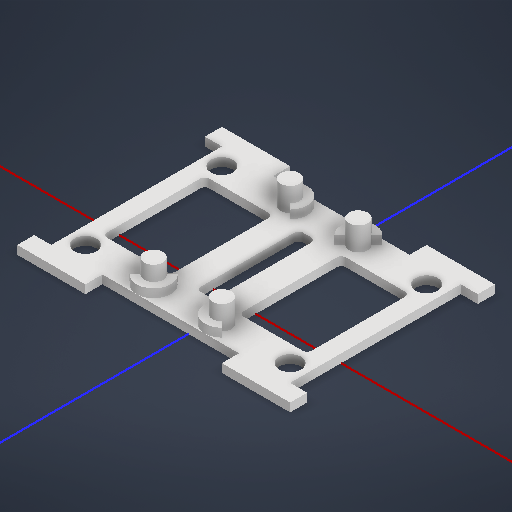
# Autodesk Inventor part: base
Saved by Autodesk Inventor 2025.4 (Build 294407000, 407)
## iProperties
Created: 2026-09-15
Part Number: base
Material: Generic
Document SubType Name: Sheet Metal
Designer: User
Density: 1 g/cm^3
Appearance: Default
Sheet Metal Rule: Default
Author: User
Autodesk Inventor part; units mm, degrees
ref_plane "YZ Plane" through (0, 0, 0) normal (1, 0, 0) x (0, 1, 0)
ref_plane "XZ Plane" through (0, 0, 0) normal (0, 1, 0) x (-1, 0, 0)
ref_plane "XY Plane" through (0, 0, 0) normal (0, 0, 1) x (1, 0, 0)
sketch "Sketch1" plane through (0, 0, 0) normal (0, 1, 0) x (-1, 0, 0)
  line L0 (-10, -14) -> (10, -14)
  line L1 (10, -14) -> (10, 14)
  line L2 (10, 14) -> (-10, 14)
  line L3 (-10, 14) -> (-10, -14)
  line L4 (-10, -14) -> (10, 14) construction
  line L5 (10, -14) -> (-10, 14) construction
  line L6 (-8, -4) -> (8, -4)
  line L7 (8, -4) -> (8, 4)
  line L8 (8, 4) -> (-8, 4)
  line L9 (-8, 4) -> (-8, -4)
  line L10 (-8, -4) -> (8, 4) construction
  line L11 (8, -4) -> (-8, 4) construction
  line L12 (-10, 8) -> (-12, 8)
  line L13 (-12, 8) -> (-12, 16)
  line L14 (-12, 16) -> (-10, 16)
  line L15 (-10, 16) -> (-10, 8)
  line L16 (10, 8) -> (12, 8)
  line L17 (12, 8) -> (12, 16)
  line L18 (12, 16) -> (10, 16)
  line L19 (10, 16) -> (10, 8)
  line L20 (10, -8) -> (12, -8)
  line L21 (12, -8) -> (12, -16)
  line L22 (12, -16) -> (10, -16)
  line L23 (10, -16) -> (10, -8)
  line L24 (-10, -8) -> (-12, -8)
  line L25 (-12, -8) -> (-12, -16)
  line L26 (-12, -16) -> (-10, -16)
  line L27 (-10, -16) -> (-10, -8)
  circle A0 centre (-8, 4) radius 2
  circle A1 centre (8, -4) radius 2
  circle A2 centre (-8, -4) radius 2
  circle A3 centre (8, 4) radius 2
  line L28 (5.5, -4) -> (-5.5, -4)
  line L29 (-6, -4.5) -> (-6, -11.5)
  line L30 (-5.5, -12) -> (5.5, -12)
  line L31 (6, -11.5) -> (6, -4.5)
  arc A4 (5.5, -12) -> (6, -11.5) centre (5.5, -11.5) ccw
  arc A5 (6, -4.5) -> (5.5, -4) centre (5.5, -4.5) ccw
  arc A6 (-6, -11.5) -> (-5.5, -12) centre (-5.5, -11.5) ccw
  arc A7 (-5.5, -4) -> (-6, -4.5) centre (-5.5, -4.5) ccw
  line L32 (5.5, 4) -> (-5.5, 4)
  line L33 (-6, 4.5) -> (-6, 11.5)
  line L34 (-5.5, 12) -> (5.5, 12)
  line L35 (6, 11.5) -> (6, 4.5)
  arc A8 (5.5, 4) -> (6, 4.5) centre (5.5, 4.5) ccw
  arc A9 (-6, 4.5) -> (-5.5, 4) centre (-5.5, 4.5) ccw
  arc A10 (6, 11.5) -> (5.5, 12) centre (5.5, 11.5) ccw
  arc A11 (-5.5, 12) -> (-6, 11.5) centre (-5.5, 11.5) ccw
  line L36 (5.5, 1) -> (-5.5, 1)
  line L37 (-6, 0.5) -> (-6, -0.5)
  line L38 (-5.5, -1) -> (5.5, -1)
  line L39 (6, -0.5) -> (6, 0.5)
  line L40 (6, 1) -> (-6, -1) construction
  line L41 (-6, 1) -> (6, -1) construction
  arc A12 (-5.5, 1) -> (-6, 0.5) centre (-5.5, 0.5) ccw
  arc A13 (-6, -0.5) -> (-5.5, -1) centre (-5.5, -0.5) ccw
  arc A14 (5.5, -1) -> (6, -0.5) centre (5.5, -0.5) ccw
  arc A15 (6, 0.5) -> (5.5, 1) centre (5.5, 0.5) ccw
  circle A16 centre (-8, 12) radius 1.3
  circle A17 centre (8, 12) radius 1.3
  circle A18 centre (-8, -12) radius 1.3
  circle A19 centre (8, -12) radius 1.3
  line L42 (-8.5858, -5.4142) -> (-4.5858, -5.4142) construction
  line L43 (11.4142, -2.5858) -> (15.4142, -2.5858) construction
  line L44 (11.4142, 2.5858) -> (15.4142, 2.5858) construction
  line L45 (-8.5858, 5.4142) -> (-4.5858, 5.4142) construction
  point P0 (0, 0)
  point P1 (-10, -14)
  point P2 (10, 4)
  point P3 (-10, 4)
  point P4 (-10, -4)
  point P5 (10, -4)
  point P6 (6, -4)
  point P7 (-6, -12)
  point P8 (-6, -4)
  point P9 (6, -12)
  point P10 (6, 4)
  point P11 (-6, 12)
  point P12 (-6, 4)
  point P13 (6, 12)
  point P14 (-5.5, 4)
  point P15 (-14.5, 16)
  point P16 (10.5, 16)
  point P17 (14.3, -16)
  point P18 (-12.7, -16)
  point P19 (12, -11)
  point P20 (12, 7)
  point P21 (-12, -6.8)
  point P22 (-12, 8.8)
  dimension "d45" = 4
  dimension "d47" = 4
  dimension "d0" = 20
  dimension "d1" = 28
  dimension "d2" = 16
  dimension "d3" = 8
  dimension "d33" = 8
  dimension "d34" = 2
  dimension "d37" = 2
  dimension "d38" = 2
  dimension "d40" = 2
  dimension "d43" = 2
  dimension "d44" = 4
  dimension "d46" = 4
  dimension "d54" = 12
  dimension "d55" = 8
  dimension "d56" = 0.5
  dimension "d57" = 12
  dimension "d58" = 8
  dimension "d59" = 0.5
  dimension "d60" = 0.5
  dimension "d61" = 12
  dimension "d62" = 2
  dimension "d63" = 0.5
  dimension "d93" = 2.6
  dimension "d94" = 2
  dimension "d96" = 2
  dimension "d97" = 2.6
  dimension "d98" = 2
  dimension "d99" = 2
  dimension "d100" = 2.6
  dimension "d101" = 2
  dimension "d102" = 2
  dimension "d103" = 2.6
  dimension "d104" = 2
  dimension "d105" = 2
  constraints: 92 end point, 38 point on line, 24 point on circle, 24 tangent, 18 centre point, 18 parallel, 13 horizontal, 9 perpendicular, 8 equal radius, 6 equal length, 6 midpoint, 4 coincident, 6 other
  measures "d0" distance of L2.end L1.end
  measures "d1" distance of L1.end L0.end
  measures "d2" distance of L8.end L7.end
  measures "d3" distance of L7.end L6.end
  measures "d33" distance of L12.end L13.end
  measures "d34" distance between parallel lines of L2 L14
  measures "d37" distance between parallel lines of L2 L18
  measures "d38" distance of L21.end L22.end
  measures "d40" distance between parallel lines of L0 L22
  measures "d43" distance between parallel lines of L0 L26
  measures "d44" diameter of A0
  measures "d46" diameter of A2
  measures "d54" distance of point (6, -12) point (-6, -12)
  measures "d55" distance of point (-6, -12) point (-6, -4)
  measures "d56" radius of A4
  measures "d57" distance of point (-6, 12) point (6, 12)
  measures "d58" distance of point (-6, 4) point (-6, 12)
  measures "d59" radius of A8
  measures "d60" radius of A10
  measures "d61" distance of L41.end L40.end
  measures "d62" distance of L40.end L41.start
  measures "d63" radius of A12
  measures "d93" diameter of A16
  measures "d94" distance from line of L2 A16.centre
  measures "d96" distance from line of L3 A16.centre
  measures "d97" diameter of A17
  measures "d98" distance from line of L2 A17.centre
  measures "d99" distance from line of L1 A17.centre
  measures "d100" diameter of A18
  measures "d101" distance from line of L3 A18.centre
  measures "d102" distance from line of L0 A18.centre
  measures "d103" diameter of A19
  measures "d104" distance from line of L1 A19.centre
  measures "d105" distance from line of L0 A19.centre
extrude "Extrusion1" add sketch "Sketch1" along normal blind 1 contours L3 A2 L6 A7 L29 A6 L30 A4 L31 A5 A1 L1 L0 | L27 L26 L25 L24 L3 | L1 L20 L21 L22 L23 | L3 A0 L9 A2 | A1 L7 A3 L1 | L3 L2 L1 A3 L8 A8 L35 A10 L34 A11 L33 A9 A0 | L9 A0 L8 A3 L7 A1 L6 A2 | L12 L13 L14 L15 L3 | L1 L19 L18 L17 L16
sketch "Sketch2" plane through (0, 0, 0) normal (0, -1, 0) x (1, 0, 0)
  line L0 (10, -14) -> (-10, -14) projected
  line L1 (10, -4) -> (10, -8) projected
  line L2 (-10, 14) -> (10, 14) projected
  line L3 (-12, -8) -> (-10, -8) projected
  line L4 (-12, -16) -> (-12, -8) projected
  line L5 (-10, -16) -> (-12, -16) projected
  line L6 (-10, 4) -> (-10, 8) projected
  line L7 (12, -16) -> (10, -16) projected
  line L8 (12, -8) -> (12, -16) projected
  line L9 (10, -8) -> (12, -8) projected
  line L10 (12, 8) -> (10, 8) projected
  line L11 (12, 16) -> (12, 8) projected
  line L12 (10, 16) -> (12, 16) projected
  line L13 (10, -16) -> (10, -14) projected
  line L14 (-10, 16) -> (-10, 14) projected
  line L15 (-12, 16) -> (-10, 16) projected
  line L16 (-12, 8) -> (-12, 16) projected
  line L17 (-10, 8) -> (-12, 8) projected
  circle A0 centre (-8, 4) radius 2 projected
  line L18 (-10, -4) -> (-10, 4) projected
  circle A1 centre (-8, -4) radius 2 projected
  line L19 (-10, -8) -> (-10, -4) projected
  circle A2 centre (8, -4) radius 2 projected
  line L20 (10, 4) -> (10, -4) projected
  circle A3 centre (8, 4) radius 2 projected
  line L21 (10, 8) -> (10, 4) projected
  line L22 (10, 14) -> (10, 16) projected
  line L23 (-10, -14) -> (-10, -16) projected
  point P0 (0, 0)
  constraints: 4 horizontal alignment
extrude "Extrusion2" add sketch "Sketch2" against normal blind 2 contours A2 | A3 | A0 | A1
sketch "Sketch3" plane through (8, 2, 4) normal (0, 1, 0) x (1, 0, 0)
  circle A0 centre (-16, 8) radius 2 projected
  circle A1 centre (0, 8) radius 2 projected
  circle A2 centre (0, 0) radius 2 projected
  circle A3 centre (-16, 0) radius 2 projected
  circle A4 centre (-16, 8) radius 1.1
  circle A5 centre (0, 8) radius 1.1
  circle A6 centre (0, 0) radius 1.1
  circle A7 centre (-16, 0) radius 1.1
  point P0 (-8, 4)
  dimension "d48" = 2.2
  dimension "d49" = 2.2
  dimension "d50" = 2.2
  dimension "d51" = 2.2
  constraints: 4 centre point, 4 coincident
  measures "d48" diameter of A4
  measures "d49" diameter of A5
  measures "d50" diameter of A6
  measures "d51" diameter of A7
extrude "Extrusion3" add sketch "Sketch3" along normal blind 1.75 contours A4 | A5 | A6 | A7
sketch "Sketch4" plane through (-8, 2, -4) normal (0, 1, 0) x (1, 0, 0)
  circle A0 centre (0, 0) radius 1.1 projected
  circle A1 centre (0, 0) radius 2 projected
  circle A2 centre (0, -8) radius 1.1 projected
  circle A3 centre (0, -8) radius 2 projected
  circle A4 centre (16, -8) radius 2 projected
  circle A5 centre (16, 0) radius 2 projected
  line L0 (-1.4142, 1.4142) -> (1.4142, -1.4142)
  line L1 (-1.4142, 1.4142) -> (2.5858, 1.4142) construction
  line L2 (14.5858, -1.4142) -> (17.4142, 1.4142)
  line L3 (14.5858, -1.4142) -> (18.5858, -1.4142) construction
  circle A6 centre (16, -8) radius 1.1 projected
  line L4 (14.5858, -6.5858) -> (17.4142, -9.4142)
  line L5 (14.5858, -6.5858) -> (18.5858, -6.5858) construction
  line L6 (-1.4142, -9.4142) -> (1.4142, -6.5858)
  line L7 (-1.4142, -9.4142) -> (2.5858, -9.4142) construction
  circle A7 centre (16, 0) radius 1.1 projected
  point P0 (8, -4)
  point P1 (16.7778, -8.7778)
  point P2 (15.2222, -7.2222)
  point P3 (14.5858, -1.4142)
  point P4 (-0.7778, 0.7778)
  point P5 (0.7778, -0.7778)
  point P6 (-1.4142, -9.4142)
  point P7 (-0.7778, -8.7778)
  point P8 (0.7778, -7.2222)
  point P9 (16.7778, 0.7778)
  point P10 (15.2222, -0.7778)
  dimension "d2" = 16
  dimension "d110" = 45
  dimension "d111" = 45
  dimension "d112" = 45
  dimension "d113" = 45
  constraints: 16 end point, 4 equal length, 4 horizontal, 4 midpoint, 8 other
  measures "d110" angle of L0 L1
  measures "d111" angle of L3 L2
  measures "d112" angle of L4 L5
  measures "d113" angle of L7 L6
extrude "Extrusion4" cut sketch "Sketch4" against normal blind 1 contours A0 L0 A1 | A2 L6 A3 | L4 A6 A4 | L2 A7 A5 | A7 L2 picked at (1.6714, 0.2412) picked at (1.569, -8.6248) picked at (14.3181, -8.146) picked at (14.402, 0.5443) picked at (15.8084, -0.3126)
move or copy body "Move Body1" bodies to move or copy 1 copy no rotation origin (0, 0, 0) rotation axis (0, 1, 0) rotation angle 90 translate (28, 0, -4)
move or copy body "Move Body2" bodies to move or copy 1 copy no translate (-30, 0, 0)
equation "\"d47\" = d45"
equation "\"d44\" = d45"
equation "\"d46\" = d45"
equation "\"d49\" = d48"
equation "\"d50\" = d48"
equation "\"d51\" = d48"
body "Solid1"
